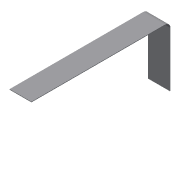
# Autodesk Inventor part: PIElectrodes
Saved by Autodesk Inventor 2014 (Build 180170000, 170)
## iProperties
Created: 2016-07-07
Part Number: PIElectrodes
Material: Generic
Document SubType Name: Modeling
Designer: Camilo
Density: 1 g/cm^3
Appearance: Default
Author: Camilo
Autodesk Inventor part; units mm, degrees
note: some values were not read from the file. Chosen so that the rebuilt part matches the saved one: bend side of "Bend Part1".
ref_plane "YZ Plane" through (0, 0, 0) normal (1, 0, 0) x (0, 1, 0)
ref_plane "XZ Plane" through (0, 0, 0) normal (0, 1, 0) x (-1, 0, 0)
ref_plane "XY Plane" through (0, 0, 0) normal (0, 0, 1) x (1, 0, 0)
sketch "Sketch1" plane through (0, 0, 0) normal (0, 1, 0) x (-1, 0, 0)
  line L0 (-2, 18) -> (-2, -18)
  line L1 (-2, -18) -> (2, -18)
  line L2 (2, -18) -> (2, 18)
  line L3 (2, 18) -> (-2, 18)
  line L4 (-2, 18) -> (2, -18) construction
  line L5 (-2, -18) -> (2, 18) construction
  point P0 (0, 0)
  constraints: 12 end point, 2 midpoint
extrude "Extrusion1" add sketch "Sketch1" along normal blind 0.1
sketch "Sketch2" plane through (0, 0.1, 0) normal (0, 1, 0) x (1, 0, 0)
  line L0 (2, -18) -> (2, 18) projected
  line L1 (2, 18) -> (-2, 18) projected
  line L2 (-2, 18) -> (-2, -18) projected
  line L3 (-2, 8) -> (2, 8)
  point P0 (0, 0)
  dimension "d2" = 10
  constraints: 2 end point, 2 point on line
  measures "d2" distance between parallel lines of L3 L1
bend part "Bend Part1" radius 1 angle 90 line through (-2, 0.1, -8) along (1, 0, 0) centre toward (0, -1, 0) moving side (0, 0, 1) both sides no
body "Solid1"
